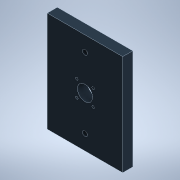
# Autodesk Inventor part: Soporte Pistón
Saved by Autodesk Inventor 2021 (Build 250183000, 183)
## iProperties
Created: 2021-05-02
Part Number: Soporte Pistón
Material: Generic
Document SubType Name: Modeling
Designer: maaro
Density: 1 g/cm^3
Appearance: Default(1)
Author: maaro
Autodesk Inventor part; units mm, degrees
ref_plane "YZ Plane" through (0, 0, 0) normal (1, 0, 0) x (0, 1, 0)
ref_plane "XZ Plane" through (0, 0, 0) normal (0, 1, 0) x (-1, 0, 0)
ref_plane "XY Plane" through (0, 0, 0) normal (0, 0, 1) x (1, 0, 0)
ref_plane "Work Plane1" through (0, 0, 0) normal (0, 0, 1) x (1, 0, 0)
sketch "Sketch1" plane through (0, 0, 0) normal (0, 0, 1) x (1, 0, 0)
  line L0 (-75, -117.1) -> (75, -117.1) projected
  line L1 (75, -117.1) -> (75, 82.9) projected
  line L2 (75, 82.9) -> (-75, 82.9) projected
  line L3 (-75, 82.9) -> (-75, -117.1) projected
  point P0 (0, -17.1)
  dimension "d11" = 100
  measures "d11" distance from line of L2 point (0, -17.1)
extrude "Extrusion1" add sketch "Sketch1" along normal blind 20
sketch "Sketch2" plane through (0, 0, 20) normal (0, 0, 1) x (1, 0, 0)
  circle A0 centre (0, -17.1) radius 15
  line L0 (75, 82.9) -> (-75, 82.9) projected
  line L1 (-75, 82.9) -> (-75, -117.1) projected
  circle A1 centre (-16.25, -0.85) radius 2.5
  circle A2 centre (16.25, -0.85) radius 2.5
  circle A3 centre (-16.25, -33.35) radius 2.5
  circle A4 centre (16.25, -33.35) radius 2.5
  point P0 (0, 0)
  dimension "d6" = 30
  dimension "d7" = 100
  dimension "d8" = 75
  dimension "d15" = 5
  dimension "d16" = 16.25
  dimension "d17" = 16.25
  dimension "d18" = 16.25
  dimension "d19" = 16.25
  dimension "d20" = 16.25
  dimension "d21" = 16.25
  dimension "d22" = 16.25
  dimension "d23" = 16.25
  constraints: 5 centre point, 3 equal radius
  measures "d6" diameter of A0
  measures "d7" distance from line of L0 A0.centre
  measures "d8" distance from line of L1 A0.centre
  measures "d15" diameter of A4
  measures "d16" horizontal distance of A0.centre A1.centre
  measures "d17" horizontal distance of A0.centre A1.centre
  measures "d18" horizontal distance of A0.centre A2.centre
  measures "d19" horizontal distance of A2.centre A0.centre
  measures "d20" horizontal distance of A0.centre A3.centre
  measures "d21" horizontal distance of A0.centre A3.centre
  measures "d22" horizontal distance of A0.centre A4.centre
  measures "d23" horizontal distance of A0.centre A4.centre
extrude "Extrusion2" cut sketch "Sketch2" against normal through all
sketch "Sketch4" plane through (0, 0, 0) normal (0, 0, -1) x (-1, 0, 0)
  circle A0 centre (0, -17.1) radius 15 projected
  circle A1 centre (0, 52.9) radius 8
  circle A2 centre (0, -87.1) radius 8
  point P0 (0, 0)
  dimension "d33" = 70
  dimension "d34" = 70
  dimension "d35" = 16
  constraints: 2 centre point, 2 coincident, 1 equal radius
  measures "d33" distance of A0.centre point (0, 52.9)
  measures "d34" distance of point (0, -87.1) A0.centre
  measures "d35" diameter of A1
extrude "Extrusion3" cut sketch "Sketch4" against normal blind 8 contours A1 | A2
sketch "Sketch5" plane through (0, 0, 20) normal (0, 0, 1) x (1, 0, 0)
  circle A0 centre (0, -17.1) radius 15 projected
  point P0 (0, 0)
  point P1 (0, -87.1)
  point P2 (0, 52.9)
  dimension "d38" = 70
  dimension "d39" = 70
  measures "d38" distance of A0.centre point (0, -87.1)
  measures "d39" distance of point (0, 52.9) A0.centre
hole "Hole2" at (0, -87.1, 20) at (0, 52.9, 20) direction (0, 0, -1) diameter 6.647 end through all counterbore diameter 10 counterbore depth 6 thread size "M8x1.25" class "6H" standard "ISO Metric profile"
equation "\"d17\" = d16"
equation "\"d18\" = d16"
equation "\"d19\" = d16"
equation "\"d20\" = d16"
equation "\"d21\" = d16"
equation "\"d22\" = d16"
equation "\"d23\" = d16"
body "Solid1"
